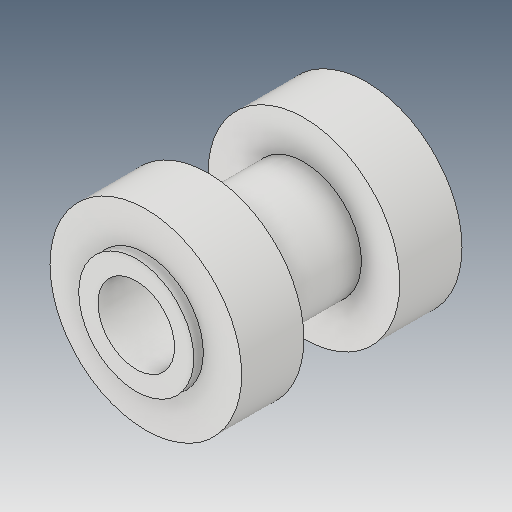
# Autodesk Inventor part: POMベアリング
Saved by Autodesk Inventor 2019.4 (Build 234330000, 330)
## iProperties
Created: 2019-06-15
Part Number: POMベアリング
Material: アセタール樹脂、白
Document SubType Name: Modeling
Designer: AzLIer
Density: 1.425 g/cm^3
Appearance: 滑らか - 白
Mass: 5.96306 g
Surface Area: 28.2743 cm^2
Volume: 4.1846 cm^3
Author: AzLIer
Autodesk Inventor part; units mm, degrees
ref_plane "YZ Plane" through (0, 0, 0) normal (1, 0, 0) x (0, 1, 0)
ref_plane "XZ Plane" through (0, 0, 0) normal (0, 1, 0) x (-1, 0, 0)
ref_plane "XY Plane" through (0, 0, 0) normal (0, 0, 1) x (1, 0, 0)
sketch "スケッチ2" plane through (0, 0, 0) normal (0, 1, 0) x (-1, 0, 0)
  line L0 (-6, 0) -> (-6, 5)
  line L1 (-6, 5) -> (-10, 5)
  line L2 (-10, 5) -> (-10, 11.5)
  line L3 (-10, 11.5) -> (-6, 11.5)
  line L4 (-6, 11.5) -> (-6, 12.5)
  line L5 (-6, 12.5) -> (-4, 12.5)
  line L6 (-4, 12.5) -> (-4, 0)
  line L7 (-4, 0) -> (-6, 0)
  line L8 (0, -14.5) -> (0, 17) projected
  circle A0 centre (0, 0) radius 4 construction
  circle A1 centre (0, 0) radius 10 construction
  circle A2 centre (0, 0) radius 6.7 construction
  dimension "d4" = 4
  dimension "d5" = 6
  dimension "d6" = 10
  dimension "d7" = 12.5
  dimension "d8" = 5
  dimension "d9" = 1
  dimension "d11" = 8
  dimension "d12" = 20
  dimension "d14" = 3.3
  constraints: 16 end point, 6 perpendicular, 3 centre point, 3 point on line, 2 coincident, 1 vertical
  measures "d4" distance from line of point (0, 0) L6
  measures "d5" distance from line of point (0, 0) L0
  measures "d6" distance from line of point (0, 0) L2
  measures "d7" distance between parallel lines of L7 L5
  measures "d8" distance between parallel lines of L7 L1
  measures "d9" distance between parallel lines of L5 L3
  measures "d11" diameter of A0
  measures "d12" diameter of A1
  measures "d14" radial gap between concentric circles of A1 A2
revolve "回転1" add sketch "スケッチ2" angle 360 about axis through (0, 0, -10) along (0, 0, 1)
mirror "ミラー1" about plane through (6, 0, 0) normal (0, 0, -1) of "回転1"
